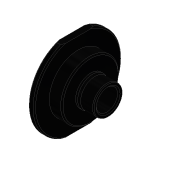
# Autodesk Inventor part: NA-45-h-Crown-247
Saved by Autodesk Inventor 2020.2 (Build 242310000, 310)
## iProperties
Created: 2020-04-21
Part Number: NA-45-h-Crown-247
Material: 12 060.4
Description: TRN
Document SubType Name: Modeling
Designer: Jurek
Density: 7.85 g/cm^3
Appearance: Eloxovaná – černá
Mass: 206.836 g
Surface Area: 123.656 cm^2
Volume: 26.3486 cm^3
User Status: Rychlá změna
Checked By: Pippal
Category: B
Hmotnost (kg): 0,21
Rozmer_A: 70
Rozmer_B: 0
Rozmer_C: 0
Rozmer_D: 29
Rada vyrobku: 4100
Prumer nadobky: 45
Cislo artiklu: 4451101360
Jednotka: ks
Cisty rozmer: =Ø<Rozmer_A> - <Rozmer_D>
Predpona: Ø
Stroj na lince: Stahovací lis
RAZ Poznamka 1: ISO 2768-mH
RAZ Poznamka 2: NEOZNAČENÉ HRANY OJEHLIT
RAZ Poznamka 3: KALIT NA 40 - 42 HRc
DXF: Ne
QAD_code: M
Rizeni davek: L
Author: Jurek
Revision Number: 00
Autodesk Inventor part; units mm, degrees
ref_plane "YZ Plane" through (0, 0, 0) normal (1, 0, 0) x (0, 1, 0)
ref_plane "XZ Plane" through (0, 0, 0) normal (0, 1, 0) x (-1, 0, 0)
ref_plane "XY Plane" through (0, 0, 0) normal (0, 0, 1) x (1, 0, 0)
sketch "Náčrt1" plane through (0, 0, 0) normal (0, 0, 1) x (1, 0, 0)
  line L0 (0, 0) -> (16.9868, 0)
  line L1 (0, 17.5) -> (0, 35)
  line L2 (5, 23) -> (15, 23)
  line L3 (15, 23) -> (15, 12)
  line L4 (15, 12) -> (16.634, 12)
  line L5 (16.634, 12) -> (18.5, 11.5)
  line L6 (18.5, 11.5) -> (29, 11.5)
  line L7 (29, 11.5) -> (29, 8.5)
  line L8 (29, 8.5) -> (11, 8.5)
  line L9 (11, 8.5) -> (11, 17.5)
  line L10 (11, 17.5) -> (0, 17.5)
  line L11 (0, 35) -> (5, 35)
  line L12 (5, 35) -> (5, 23)
  dimension "d0" = 29
  dimension "d2" = 10.5
  dimension "d5" = 14
  dimension "d8" = 46
  dimension "d10" = 24
  dimension "d11" = 23
  dimension "d12" = 17
  dimension "d13" = 35
  dimension "d14" = 11
  dimension "d15" = 15
  dimension "d40" = 12.366
  dimension "d53" = 70
  dimension "d54" = 24
  constraints: 26 end point, 4 perpendicular, 3 parallel, 1 horizontal, 1 point on line
  measures "d0" distance between parallel lines of L7 L1
  measures "d2" distance from line of L5.end L7
  measures "d5" distance between parallel lines of L3 L7
  measures "d8" diameter of L2 L0
  measures "d10" diameter of L4 L0
  measures "d11" diameter of L6 L0
  measures "d12" diameter of L8 L0
  measures "d13" diameter of L10 L0
  measures "d14" distance between parallel lines of L9 L1
  measures "d15" angle of L5 L4
  measures "d40" distance from line of L4.end L7
  measures "d53" diameter of L11 L0
  measures "d54" distance between parallel lines of L12 L7
revolve "Rotace1" add sketch "Náčrt1" angle 360 about axis through (0, 0, 0) along (1, 0, 0)
chamfer "Zkosení3" distance 1 angle 45 1 edges at (15, -23, 0)
chamfer "Zkosení5" distance 1 angle 15 1 edges at (29, -11.5, 0) measured on face at (25.5, 11.4627, -0.9254)
chamfer "Zkosení6" distance 0.5 angle 45 1 edges at (0, -17.5, 0)
chamfer "Zkosení8" distance 1 angle 45 1 edges at (29, -8.5, 0)
chamfer "Zkosení9" distance 1 angle 45 1 edges at (11, -8.5, 0)
chamfer "Zkosení11" distance 1 angle 45 1 edges at (5, -35, 0)
chamfer "Zkosení12" distance 1 angle 45 1 edges at (0, -35, 0)
sketch "Náčrt3" plane through (0, 0, 0) normal (-1, 0, 0) x (0, 0, 1)
  line L0 (-39.3312, 12.9904) -> (-32.5, 12.9904)
  line L1 (-32.5, 12.9904) -> (-32.5, -12.9904)
  line L2 (-32.5, -12.9904) -> (-39.3312, -12.9904)
  line L3 (-39.3312, -12.9904) -> (-39.3312, 12.9904)
  line L4 (52.9331, 12.9904) -> (32.5, 12.9904)
  line L5 (32.5, 12.9904) -> (32.5, -12.9904)
  line L6 (32.5, -12.9904) -> (52.9331, -12.9904)
  line L7 (52.9331, -12.9904) -> (52.9331, 12.9904)
  line L8 (0, 0) -> (0, -6.1481) construction
  circle A0 centre (0, 0) radius 35 construction
  dimension "d61" = 65
  constraints: 18 end point, 5 parallel, 2 horizontal, 2 perpendicular, 2 point on circle, 2 point on line, 1 other
  measures "d61" distance between parallel lines of L5 L1
extrude "Vysunutí2" cut sketch "Náčrt3" against normal through all
equation "\"Rozmer_B\" = 0"
equation "\"Rozmer_C\" = 0"
equation "\"Rozmer_D\" = d0"
